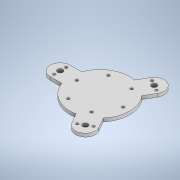
# Autodesk Inventor part: De_Mica
Saved by Autodesk Inventor 2022 (Build 260153000, 153)
## iProperties
Created: 2022-11-22
Part Number: De_Mica
Material: Generic
Document SubType Name: Modeling
Designer: nguye
Density: 1 g/cm^3
Appearance: Default
Author: nguye
Autodesk Inventor part; units mm, degrees
ref_plane "YZ Plane" through (0, 0, 0) normal (1, 0, 0) x (0, 1, 0)
ref_plane "XZ Plane" through (0, 0, 0) normal (0, 1, 0) x (-1, 0, 0)
ref_plane "XY Plane" through (0, 0, 0) normal (0, 0, 1) x (1, 0, 0)
sketch "Sketch1" plane through (0, 0, 0) normal (0, 1, 0) x (-1, 0, 0)
  circle A0 centre (0, 0) radius 75
  dimension "d0" = 150
  constraints: 1 centre point, 1 coincident
  measures "d0" diameter of A0
extrude "Extrusion1" add sketch "Sketch1" along normal blind 5
sketch "Sketch2" plane through (0, 5, 0) normal (0, 1, 0) x (1, 0, 0)
  point P0 (0, 0)
  point P1 (-60, 0)
  dimension "d4" = 60
  constraints: 1 horizontal alignment
  measures "d4" distance of point (0, 0) point (-60, 0)
hole "Hole1" at (-60, 5, 0) direction (0, -1, 0) diameter 8 end through all
pattern_circular "Circular Pattern1" count 3 over 360 about axis through (0, -10, 0) along (0, 1, 0) of "Hole1"
sketch "Sketch3" plane through (0, 5, 0) normal (0, 1, 0) x (1, 0, 0)
  circle A0 centre (-60, 0) radius 4 projected
  circle A1 centre (-60, 0) radius 15
  circle A2 centre (30, -51.9615) radius 15
  circle A3 centre (30, 51.9615) radius 15
  circle A4 centre (30, -51.9615) radius 4 projected
  circle A5 centre (0, 0) radius 60
  circle A6 centre (0, 0) radius 75 projected
  point P0 (-75, 0)
  point P1 (37.5, -64.9519)
  point P2 (16.174, -57.7789)
  point P3 (-58.125, -14.8824)
  point P4 (37.5, 64.9519)
  point P5 (41.951, 42.8966)
  point P6 (41.951, -42.8966)
  point P7 (-58.125, 14.8824)
  point P8 (16.174, 57.7789)
  dimension "d15" = 30
  dimension "d18" = 360
  constraints: 3 centre point, 2 coincident, 10 other
  measures "d15" diameter of A1
extrude "Extrusion2" cut sketch "Sketch3" against normal through all contours A1 A6 A3 A5 | A5 A2 A6 A1 | A6 A2 A5 A3
sketch "Sketch4" plane through (0, 5, 0) normal (0, 1, 0) x (1, 0, 0)
  circle A0 centre (-60, 0) radius 4 projected
  point P0 (0, 0)
  point P1 (-60, -9)
  point P2 (-60, 9)
  dimension "d22" = 18
  dimension "d23" = 9
  constraints: 2 vertical alignment
  measures "d22" distance of point (-60, 9) point (-60, -9)
  measures "d23" vertical distance of point (0, 0) point (-60, 9)
hole "Hole2" at (-60, 5, 9) at (-60, 5, -9) direction (0, -1, 0) diameter 4 end through all
pattern_circular "Circular Pattern2" count 3 over 360 about axis through (0, -10, 0) along (0, 1, 0) of "Hole2"
sketch "Sketch6" plane through (0, 5, 0) normal (0, 1, 0) x (1, 0, 0)
  circle A0 centre (0, 0) radius 45
  arc A1 (-58.125, 14.8824) -> (-58.125, -14.8824) centre (-60, 0) ccw projected
  line L0 (-60, -15) -> (-42.4264, -15)
  line L1 (-60, 15) -> (-42.4264, 15)
  arc A2 (-58.125, 14.8824) -> (-58.125, -14.8824) centre (-60, 0) ccw projected
  line L2 (42.9904, -44.4615) -> (34.2036, -29.2423)
  line L3 (17.0096, -59.4615) -> (8.2228, -44.2423)
  line L4 (17.0096, 59.4615) -> (8.2228, 44.2423)
  line L5 (42.9904, 44.4615) -> (34.2036, 29.2423)
  arc A3 (-58.125, -14.8824) -> (16.174, -57.7789) centre (0, 0) ccw projected
  arc A4 (41.951, -42.8966) -> (41.951, 42.8966) centre (0, 0) ccw projected
  circle A5 centre (22.2058, 56.4615) radius 2 projected
  circle A6 centre (37.7942, 47.4615) radius 2 projected
  circle A7 centre (37.7942, -47.4615) radius 2 projected
  circle A8 centre (22.2058, -56.4615) radius 2 projected
  circle A9 centre (-60, -9) radius 2 projected
  circle A10 centre (-60, 9) radius 2 projected
  arc A11 (-58.125, 14.8824) -> (-58.125, -14.8824) centre (-60, 0) ccw projected
  arc A12 (-58.125, -14.8824) -> (16.174, -57.7789) centre (0, 0) ccw projected
  arc A13 (16.174, -57.7789) -> (41.951, -42.8966) centre (30, -51.9615) ccw projected
  arc A14 (41.951, -42.8966) -> (41.951, 42.8966) centre (0, 0) ccw projected
  arc A15 (41.951, 42.8966) -> (16.174, 57.7789) centre (30, 51.9615) ccw projected
  arc A16 (16.174, 57.7789) -> (-58.125, 14.8824) centre (0, 0) ccw projected
  circle A17 centre (30, 51.9615) radius 4 projected
  circle A18 centre (30, -51.9615) radius 4 projected
  circle A19 centre (-60, 0) radius 4 projected
  point P0 (-58.0948, -15)
  point P1 (16.057, -57.8115)
  point P2 (16.057, 57.8115)
  point P3 (-58.0948, 15)
  point P4 (42.0378, -42.8115)
  point P5 (42.0378, 42.8115)
  point P6 (-58.125, 14.8824)
  point P7 (41.951, 42.8966)
  point P8 (16.174, -57.7789)
  dimension "d55" = 90
  dimension "d58" = 360
  constraints: 12 end point, 4 point on circle, 2 tangent, 1 centre point, 1 coincident, 1 horizontal, 1 parallel, 19 other
  measures "d55" diameter of A0
extrude "Extrusion3" cut sketch "Sketch6" against normal blind 10 contours A0 L5 A4 L2 | A0 L1 A16 L4 | L3 A3 L0 A0
sketch "Sketch7" plane through (0, 5, 0) normal (0, 1, 0) x (1, 0, 0)
  point P0 (0, 0)
  point P1 (-35, 0)
  point P2 (-17.5, -30.3109)
  point P3 (17.5, -30.3109)
  point P4 (35, 0)
  point P5 (17.5, 30.3109)
  point P6 (-17.5, 30.3109)
  dimension "d63" = 35
  dimension "d66" = 360
  constraints: 1 horizontal alignment, 7 other
  measures "d63" distance of point (0, 0) point (-35, 0)
hole "Hole4" at (-35, 5, 0) at (-17.5, 5, 30.3109) at (17.5, 5, 30.3109) at (35, 5, 0) at (17.5, 5, -30.3109) at (-17.5, 5, -30.3109) direction (0, -1, 0) diameter 4 end through all
extrude "Extrusion4" add sketch "Sketch6" against normal up to surface (5 mm away) contours A4 A15 L5 | L2 A13 A4 | L4 A15 A16 | A3 A13 L3 | A16 A1 L1 | L0 A1 A3
body "Solid1"
